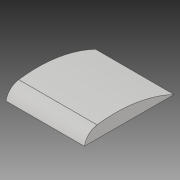
# Autodesk Inventor part: Basic
Saved by Autodesk Inventor 2018.2 (Build 222227000, 227)
## iProperties
Created: 2018-02-04
Part Number: Basic
Material: Generic
Document SubType Name: Modeling
Designer: Rus
Density: 1 g/cm^3
Appearance: Default
Author: Rus
Autodesk Inventor part; units mm, degrees
ref_plane "YZ Plane" through (0, 0, 0) normal (1, 0, 0) x (0, 1, 0)
ref_plane "XZ Plane" through (0, 0, 0) normal (0, 1, 0) x (-1, 0, 0)
ref_plane "XY Plane" through (0, 0, 0) normal (0, 0, 1) x (1, 0, 0)
sketch "Sketch1" plane through (0, 0, 0) normal (1, 0, 0) x (0, 1, 0)
  line L0 (0, 0) -> (0, -50.8)
  arc A0 (6.9175, -7.1843) -> (0, 0) centre (-1.4702, -8.338) ccw
  arc A1 (0, -50.8) -> (6.9175, -7.1843) centre (-68.5717, -17.5681) ccw
  line L1 (0, 0) -> (-73.5094, 12.9617) construction
  dimension "d0" = 100
  dimension "d1" = 50.8
  dimension "d2" = 8.4667
  dimension "d3" = 76.2
  constraints: 4 end point, 4 point on circle, 2 centre point, 2 tangent, 1 vertical
  measures "d0" angle of L1 L0
  measures "d1" distance of L0.start L0.end
  measures "d2" radius of A0
  measures "d3" radius of A1
extrude "Extrusion1" add sketch "Sketch1" along normal mid plane 44.45
body "Solid1"
